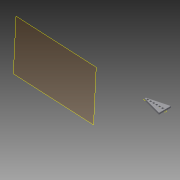
# Autodesk Inventor part: brace01
Saved by Autodesk Inventor 2013 (Build 170138000, 138)
## iProperties
Created: 2013-02-22
Part Number: brace01
Material: Generic
Document SubType Name: Modeling
Designer: Nano
Density: 1 g/cm^3
d15: 6.000 ul
d17: 0.500 in
d22: 0.250 in
d23: 0.00 deg
Author: Nano
Autodesk Inventor part; units mm, degrees
ref_plane "YZ Plane" through (0, 0, 0) normal (1, 0, 0) x (0, 1, 0)
ref_plane "XZ Plane" through (0, 0, 0) normal (0, 1, 0) x (-1, 0, 0)
ref_plane "XY Plane" through (0, 0, 0) normal (0, 0, 1) x (1, 0, 0)
ref_plane "Work Plane1" through (-521.128, -68.463, 0) normal (0, 0, 1) x (-0.9986, 0.0523, 0)
ref_plane "Work Plane2" through (223.5893, -43.1165, -6.351) normal (0, -1, 0) x (1, 0, 0)
sketch "Sketch1" plane through (223.5893, -43.1165, -6.351) normal (0, -1, 0) x (1, 0, 0)
  line L0 (-282.6219, 6.351) -> (-282.6219, 0.001) projected
  line L1 (-173.8519, 0.001) -> (-282.6219, 0.001) projected
  line L2 (-282.6219, 6.351) -> (-173.8519, 6.351) projected
  line L3 (-283.1206, 28.576) -> (-366.4496, 6.351)
  line L4 (-283.1206, 3.176) -> (-376.14, 3.176) construction
  line L5 (-283.1206, -22.224) -> (-366.4496, 0.001)
  line L6 (-366.4496, 6.351) -> (-366.4496, 0.001)
  line L7 (-283.1206, 28.576) -> (-283.1206, -22.224)
  line L8 (-289.4706, 0.001) -> (-295.8206, 0.001)
  line L9 (-295.8206, 0.001) -> (-295.8206, 6.351)
  line L10 (-295.8206, 6.351) -> (-289.4706, 6.351)
  line L11 (-289.4706, 6.351) -> (-289.4706, 0.001)
  line L12 (-302.1706, 0.001) -> (-308.5206, 0.001)
  line L13 (-308.5206, 0.001) -> (-308.5206, 6.351)
  line L14 (-308.5206, 6.351) -> (-302.1706, 6.351)
  line L15 (-302.1706, 6.351) -> (-302.1706, 0.001)
  line L16 (-314.8706, 0.001) -> (-321.2206, 0.001)
  line L17 (-321.2206, 0.001) -> (-321.2206, 6.351)
  line L18 (-321.2206, 6.351) -> (-314.8706, 6.351)
  line L19 (-314.8706, 6.351) -> (-314.8706, 0.001)
  line L20 (-327.5706, 0.001) -> (-333.9206, 0.001)
  line L21 (-333.9206, 0.001) -> (-333.9206, 6.351)
  line L22 (-333.9206, 6.351) -> (-327.5706, 6.351)
  line L23 (-327.5706, 6.351) -> (-327.5706, 0.001)
  line L24 (-340.2706, 0.001) -> (-346.6206, 0.001)
  line L25 (-346.6206, 0.001) -> (-346.6206, 6.351)
  line L26 (-346.6206, 6.351) -> (-340.2706, 6.351)
  line L27 (-340.2706, 6.351) -> (-340.2706, 0.001)
  line L28 (-352.9706, 0.001) -> (-359.3206, 0.001)
  line L29 (-359.3206, 0.001) -> (-359.3206, 6.351)
  line L30 (-359.3206, 6.351) -> (-352.9706, 6.351)
  line L31 (-352.9706, 6.351) -> (-352.9706, 0.001)
  line L32 (-282.6219, 6.351) -> (-282.6219, 0.001) projected
  line L33 (-173.8519, 6.351) -> (-173.8519, 0.001) projected
  point P0 (-223.5893, 6.351)
  dimension "d17" = 12.7
  constraints: 58 end point, 2 horizontal, 2 parallel, 2 symmetric about line, 1 perpendicular, 40 other
  measures "d17" distance of L8.start L12.start
extrude "Extrusion2" add sketch "Sketch1" against normal blind 6.35 contours L7 L5 L6 L3
body "Solid2"
